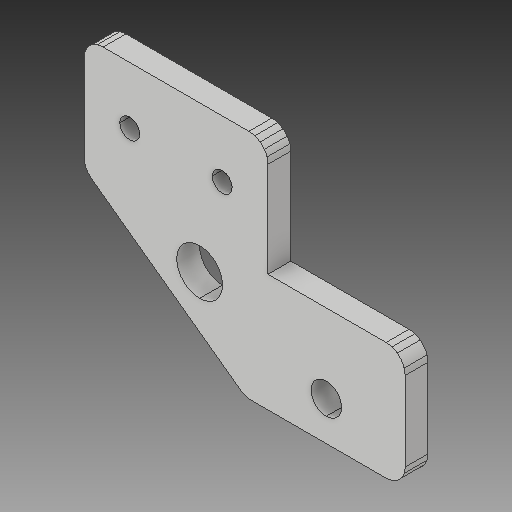
# Autodesk Inventor part: Leadscrew-rod-holder
Saved by Autodesk Inventor 2018 (Build 220112000, 112)
## iProperties
Created: 2016-07-23
Part Number: Leadscrew-rod-holder
Material: Generic
Document SubType Name: Modeling
Designer: joshm_000
Density: 1 g/cm^3
Appearance: Default
Author: joshm_000
Autodesk Inventor part; units mm, degrees
ref_plane "YZ Plane" through (0, 0, 0) normal (1, 0, 0) x (0, 1, 0)
ref_plane "XZ Plane" through (0, 0, 0) normal (0, 1, 0) x (-1, 0, 0)
ref_plane "XY Plane" through (0, 0, 0) normal (0, 0, 1) x (1, 0, 0)
sketch "Sketch1" plane through (0, 0, 0) normal (0, 0, 1) x (1, 0, 0)
  line L0 (83.1982, 140.877) -> (83.1982, 118.4214)
  spline S0 degree 3 poles (83.1982, 118.4214) (83.1982, 117.8956) (83.2805, 117.3761) (83.443, 116.8762) knots 1 1 1 1 2 2 2 2
  line L1 (83.1982, 118.4214) -> (83.1982, 117.8956) construction
  line L2 (83.1982, 117.8956) -> (83.2805, 117.3761) construction
  line L3 (83.2805, 117.3761) -> (83.443, 116.8762) construction
  spline S1 degree 3 poles (83.443, 116.8762) (83.6054, 116.3762) (83.8442, 115.9078) (84.1532, 115.4824) knots 2 2 2 2 3 3 3 3
  line L4 (83.443, 116.8762) -> (83.6054, 116.3762) construction
  line L5 (83.6054, 116.3762) -> (83.8442, 115.9078) construction
  line L6 (83.8442, 115.9078) -> (84.1532, 115.4824) construction
  spline S2 degree 3 poles (84.1532, 115.4824) (84.4612, 115.0586) (84.8315, 114.6879) (85.2551, 114.3792) knots 3 3 3 3 4 4 4 4
  line L7 (84.1532, 115.4824) -> (84.4612, 115.0586) construction
  line L8 (84.4612, 115.0586) -> (84.8315, 114.6879) construction
  line L9 (84.8315, 114.6879) -> (85.2551, 114.3792) construction
  line L10 (85.2551, 114.3792) -> (124.2313, 85.9985)
  spline S3 degree 3 poles (124.2313, 85.9985) (124.6565, 85.689) (125.1247, 85.4497) (125.6245, 85.2868) knots 5 5 5 5 6 6 6 6
  line L11 (124.2313, 85.9985) -> (124.6565, 85.689) construction
  line L12 (124.6565, 85.689) -> (125.1247, 85.4497) construction
  line L13 (125.1247, 85.4497) -> (125.6245, 85.2868) construction
  spline S4 degree 3 poles (125.6245, 85.2868) (126.1262, 85.1233) (126.647, 85.0405) (127.1745, 85.0405) knots 6 6 6 6 7 7 7 7
  line L14 (125.6245, 85.2868) -> (126.1262, 85.1233) construction
  line L15 (126.1262, 85.1233) -> (126.647, 85.0405) construction
  line L16 (126.647, 85.0405) -> (127.1745, 85.0405) construction
  line L17 (127.1745, 85.0405) -> (157.5604, 85.0405)
  line L18 (157.5604, 85.0405) -> (162.48, 85.0405)
  spline S5 degree 3 poles (162.48, 85.0405) (163.0057, 85.0405) (163.5251, 85.1228) (164.0251, 85.2852) (164.5252, 85.4477) (164.9935, 85.6864) (165.419, 85.9954) knots 9 9 9 9 10 10 10 11 11 11 11
  line L19 (162.48, 85.0405) -> (163.0057, 85.0405) construction
  line L20 (163.0057, 85.0405) -> (163.5251, 85.1228) construction
  line L21 (163.5251, 85.1228) -> (164.0251, 85.2852) construction
  line L22 (164.0251, 85.2852) -> (164.5252, 85.4477) construction
  line L23 (164.5252, 85.4477) -> (164.9935, 85.6864) construction
  line L24 (164.9935, 85.6864) -> (165.419, 85.9954) construction
  spline S6 degree 3 poles (165.419, 85.9954) (165.8443, 86.3045) (166.216, 86.6762) (166.5251, 87.1017) knots 11 11 11 11 12 12 12 12
  line L25 (165.419, 85.9954) -> (165.8443, 86.3045) construction
  line L26 (165.8443, 86.3045) -> (166.216, 86.6762) construction
  line L27 (166.216, 86.6762) -> (166.5251, 87.1017) construction
  spline S7 degree 3 poles (166.5251, 87.1017) (166.8341, 87.5268) (167.0728, 87.9953) (167.2353, 88.4955) knots 12 12 12 12 13 13 13 13
  line L28 (166.5251, 87.1017) -> (166.8341, 87.5268) construction
  line L29 (166.8341, 87.5268) -> (167.0728, 87.9953) construction
  line L30 (167.0728, 87.9953) -> (167.2353, 88.4955) construction
  spline S8 degree 3 poles (167.2353, 88.4955) (167.3977, 88.9954) (167.48, 89.5146) (167.48, 90.0403) knots 13 13 13 13 14 14 14 14
  line L31 (167.2353, 88.4955) -> (167.3977, 88.9954) construction
  line L32 (167.3977, 88.9954) -> (167.48, 89.5146) construction
  line L33 (167.48, 89.5146) -> (167.48, 90.0403) construction
  line L34 (167.48, 90.0403) -> (167.48, 110.877)
  spline S9 degree 3 poles (167.48, 110.877) (167.48, 111.4027) (167.3977, 111.9219) (167.2353, 112.4221) knots 15 15 15 15 16 16 16 16
  line L35 (167.48, 110.877) -> (167.48, 111.4027) construction
  line L36 (167.48, 111.4027) -> (167.3977, 111.9219) construction
  line L37 (167.3977, 111.9219) -> (167.2353, 112.4221) construction
  spline S10 degree 3 poles (167.2353, 112.4221) (167.0728, 112.9221) (166.8341, 113.3905) (166.5251, 113.816) (166.216, 114.2414) (165.8443, 114.6132) (165.419, 114.9222) knots 16 16 16 16 17 17 17 18 18 18 18
  line L38 (167.2353, 112.4221) -> (167.0728, 112.9221) construction
  line L39 (167.0728, 112.9221) -> (166.8341, 113.3905) construction
  line L40 (166.8341, 113.3905) -> (166.5251, 113.816) construction
  line L41 (166.5251, 113.816) -> (166.216, 114.2414) construction
  line L42 (166.216, 114.2414) -> (165.8443, 114.6132) construction
  line L43 (165.8443, 114.6132) -> (165.419, 114.9222) construction
  spline S11 degree 3 poles (165.419, 114.9222) (164.9935, 115.2312) (164.5252, 115.47) (164.0251, 115.6322) knots 18 18 18 18 19 19 19 19
  line L44 (165.419, 114.9222) -> (164.9935, 115.2312) construction
  line L45 (164.9935, 115.2312) -> (164.5252, 115.47) construction
  line L46 (164.5252, 115.47) -> (164.0251, 115.6322) construction
  spline S12 degree 3 poles (164.0251, 115.6322) (163.5251, 115.7948) (163.0057, 115.877) (162.48, 115.877) knots 19 19 19 19 20 20 20 20
  line L47 (164.0251, 115.6322) -> (163.5251, 115.7948) construction
  line L48 (163.5251, 115.7948) -> (163.0057, 115.877) construction
  line L49 (163.0057, 115.877) -> (162.48, 115.877) construction
  line L50 (162.48, 115.877) -> (131.48, 115.877)
  line L51 (131.48, 115.877) -> (131.48, 140.877)
  spline S13 degree 3 poles (131.48, 140.877) (131.48, 141.4029) (131.3978, 141.9221) (131.2352, 142.422) knots 22 22 22 22 23 23 23 23
  line L52 (131.48, 140.877) -> (131.48, 141.4029) construction
  line L53 (131.48, 141.4029) -> (131.3978, 141.9221) construction
  line L54 (131.3978, 141.9221) -> (131.2352, 142.422) construction
  spline S14 degree 3 poles (131.2352, 142.422) (131.073, 142.9222) (130.8342, 143.3906) (130.5252, 143.8159) knots 23 23 23 23 24 24 24 24
  line L55 (131.2352, 142.422) -> (131.073, 142.9222) construction
  line L56 (131.073, 142.9222) -> (130.8342, 143.3906) construction
  line L57 (130.8342, 143.3906) -> (130.5252, 143.8159) construction
  spline S15 degree 3 poles (130.5252, 143.8159) (130.2162, 144.2413) (129.8443, 144.6131) (129.419, 144.9221) knots 24 24 24 24 25 25 25 25
  line L58 (130.5252, 143.8159) -> (130.2162, 144.2413) construction
  line L59 (130.2162, 144.2413) -> (129.8443, 144.6131) construction
  line L60 (129.8443, 144.6131) -> (129.419, 144.9221) construction
  spline S16 degree 3 poles (129.419, 144.9221) (128.9935, 145.2311) (128.5251, 145.4698) (128.0251, 145.6325) knots 25 25 25 25 26 26 26 26
  line L61 (129.419, 144.9221) -> (128.9935, 145.2311) construction
  line L62 (128.9935, 145.2311) -> (128.5251, 145.4698) construction
  line L63 (128.5251, 145.4698) -> (128.0251, 145.6325) construction
  spline S17 degree 3 poles (128.0251, 145.6325) (127.525, 145.7947) (127.0057, 145.8771) (126.48, 145.8771) knots 26 26 26 26 27 27 27 27
  line L64 (128.0251, 145.6325) -> (127.525, 145.7947) construction
  line L65 (127.525, 145.7947) -> (127.0057, 145.8771) construction
  line L66 (127.0057, 145.8771) -> (126.48, 145.8771) construction
  line L67 (126.48, 145.8771) -> (120.08, 145.8771)
  line L68 (120.08, 145.8771) -> (115.1604, 145.8771)
  line L69 (115.1604, 145.8771) -> (88.1982, 145.8771)
  spline S18 degree 3 poles (88.1982, 145.8771) (87.6723, 145.8771) (87.1532, 145.7947) (86.6533, 145.6325) knots 30 30 30 30 31 31 31 31
  line L70 (88.1982, 145.8771) -> (87.6723, 145.8771) construction
  line L71 (87.6723, 145.8771) -> (87.1532, 145.7947) construction
  line L72 (87.1532, 145.7947) -> (86.6533, 145.6325) construction
  spline S19 degree 3 poles (86.6533, 145.6325) (86.1531, 145.4698) (85.6845, 145.2311) (85.2594, 144.9221) knots 31 31 31 31 32 32 32 32
  line L73 (86.6533, 145.6325) -> (86.1531, 145.4698) construction
  line L74 (86.1531, 145.4698) -> (85.6845, 145.2311) construction
  line L75 (85.6845, 145.2311) -> (85.2594, 144.9221) construction
  spline S20 degree 3 poles (85.2594, 144.9221) (84.8339, 144.6131) (84.4622, 144.2413) (84.1532, 143.8159) knots 32 32 32 32 33 33 33 33
  line L76 (85.2594, 144.9221) -> (84.8339, 144.6131) construction
  line L77 (84.8339, 144.6131) -> (84.4622, 144.2413) construction
  line L78 (84.4622, 144.2413) -> (84.1532, 143.8159) construction
  spline S21 degree 3 poles (84.1532, 143.8159) (83.8442, 143.3906) (83.6054, 142.9222) (83.443, 142.422) knots 33 33 33 33 34 34 34 34
  line L79 (84.1532, 143.8159) -> (83.8442, 143.3906) construction
  line L80 (83.8442, 143.3906) -> (83.6054, 142.9222) construction
  line L81 (83.6054, 142.9222) -> (83.443, 142.422) construction
  spline S22 degree 3 poles (83.443, 142.422) (83.2805, 141.9221) (83.1982, 141.4029) (83.1982, 140.877) knots 34 34 34 34 35 35 35 35
  line L82 (83.443, 142.422) -> (83.2805, 141.9221) construction
  line L83 (83.2805, 141.9221) -> (83.1982, 141.4029) construction
  line L84 (83.1982, 141.4029) -> (83.1982, 140.877) construction
  spline S23 degree 3 poles (146.7912, 91.2547) (144.5819, 91.2547) (142.7911, 93.0455) (142.7911, 95.2547) (142.7911, 97.4638) (144.5819, 99.2546) (146.7912, 99.2546) (149.0002, 99.2546) (150.7911, 97.4638) (150.7911, 95.2547) (150.7911, 93.0455) (149.0002, 91.2547) (146.7912, 91.2547) knots 0 0 0 0 1 1 1 2 2 2 3 3 3 4 4 4 4
  line L85 (146.7912, 91.2547) -> (144.5819, 91.2547) construction
  line L86 (144.5819, 91.2547) -> (142.7911, 93.0455) construction
  line L87 (142.7911, 93.0455) -> (142.7911, 95.2547) construction
  line L88 (142.7911, 95.2547) -> (142.7911, 97.4638) construction
  line L89 (142.7911, 97.4638) -> (144.5819, 99.2546) construction
  line L90 (144.5819, 99.2546) -> (146.7912, 99.2546) construction
  line L91 (146.7912, 99.2546) -> (149.0002, 99.2546) construction
  line L92 (149.0002, 99.2546) -> (150.7911, 97.4638) construction
  line L93 (150.7911, 97.4638) -> (150.7911, 95.2547) construction
  line L94 (150.7911, 95.2547) -> (150.7911, 93.0455) construction
  line L95 (150.7911, 93.0455) -> (149.0002, 91.2547) construction
  line L96 (149.0002, 91.2547) -> (146.7912, 91.2547) construction
  spline S24 degree 3 poles (95.1982, 128.2771) (93.7622, 128.2771) (92.5981, 129.4412) (92.5981, 130.8771) (92.5981, 132.313) (93.7622, 133.4771) (95.1982, 133.4771) (96.6341, 133.4771) (97.7982, 132.313) (97.7982, 130.8771) (97.7982, 129.4412) (96.6341, 128.2771) (95.1982, 128.2771) knots 0 0 0 0 1 1 1 2 2 2 3 3 3 4 4 4 4
  line L97 (95.1982, 128.2771) -> (93.7622, 128.2771) construction
  line L98 (93.7622, 128.2771) -> (92.5981, 129.4412) construction
  line L99 (92.5981, 129.4412) -> (92.5981, 130.8771) construction
  line L100 (92.5981, 130.8771) -> (92.5981, 132.313) construction
  line L101 (92.5981, 132.313) -> (93.7622, 133.4771) construction
  line L102 (93.7622, 133.4771) -> (95.1982, 133.4771) construction
  line L103 (95.1982, 133.4771) -> (96.6341, 133.4771) construction
  line L104 (96.6341, 133.4771) -> (97.7982, 132.313) construction
  line L105 (97.7982, 132.313) -> (97.7982, 130.8771) construction
  line L106 (97.7982, 130.8771) -> (97.7982, 129.4412) construction
  line L107 (97.7982, 129.4412) -> (96.6341, 128.2771) construction
  line L108 (96.6341, 128.2771) -> (95.1982, 128.2771) construction
  spline S25 degree 3 poles (119.48, 128.2771) (118.044, 128.2771) (116.88, 129.4412) (116.88, 130.8771) (116.88, 132.313) (118.044, 133.4771) (119.48, 133.4771) (120.916, 133.4771) (122.0799, 132.313) (122.0799, 130.8771) (122.0799, 129.4412) (120.916, 128.2771) (119.48, 128.2771) knots 0 0 0 0 1 1 1 2 2 2 3 3 3 4 4 4 4
  line L109 (119.48, 128.2771) -> (118.044, 128.2771) construction
  line L110 (118.044, 128.2771) -> (116.88, 129.4412) construction
  line L111 (116.88, 129.4412) -> (116.88, 130.8771) construction
  line L112 (116.88, 130.8771) -> (116.88, 132.313) construction
  line L113 (116.88, 132.313) -> (118.044, 133.4771) construction
  line L114 (118.044, 133.4771) -> (119.48, 133.4771) construction
  line L115 (119.48, 133.4771) -> (120.916, 133.4771) construction
  line L116 (120.916, 133.4771) -> (122.0799, 132.313) construction
  line L117 (122.0799, 132.313) -> (122.0799, 130.8771) construction
  line L118 (122.0799, 130.8771) -> (122.0799, 129.4412) construction
  line L119 (122.0799, 129.4412) -> (120.916, 128.2771) construction
  line L120 (120.916, 128.2771) -> (119.48, 128.2771) construction
  spline S26 degree 3 poles (146.7912, 91.5045) (144.72, 91.5045) (143.0412, 93.1836) (143.0412, 95.2547) (143.0412, 97.3257) (144.72, 99.0045) (146.7912, 99.0045) (148.8622, 99.0045) (150.5412, 97.3257) (150.5412, 95.2547) (150.5412, 93.1836) (148.8622, 91.5045) (146.7912, 91.5045) knots 0 0 0 0 1 1 1 2 2 2 3 3 3 4 4 4 4
  line L121 (146.7912, 91.5045) -> (144.72, 91.5045) construction
  line L122 (144.72, 91.5045) -> (143.0412, 93.1836) construction
  line L123 (143.0412, 93.1836) -> (143.0412, 95.2547) construction
  line L124 (143.0412, 95.2547) -> (143.0412, 97.3257) construction
  line L125 (143.0412, 97.3257) -> (144.72, 99.0045) construction
  line L126 (144.72, 99.0045) -> (146.7912, 99.0045) construction
  line L127 (146.7912, 99.0045) -> (148.8622, 99.0045) construction
  line L128 (148.8622, 99.0045) -> (150.5412, 97.3257) construction
  line L129 (150.5412, 97.3257) -> (150.5412, 95.2547) construction
  line L130 (150.5412, 95.2547) -> (150.5412, 93.1836) construction
  line L131 (150.5412, 93.1836) -> (148.8622, 91.5045) construction
  line L132 (148.8622, 91.5045) -> (146.7912, 91.5045) construction
  spline S27 degree 3 poles (113.5312, 101.426) (110.2174, 101.426) (107.5312, 104.1123) (107.5312, 107.426) (107.5312, 110.7398) (110.2174, 113.426) (113.5312, 113.426) (116.8449, 113.426) (119.5312, 110.7398) (119.5312, 107.426) (119.5312, 104.1123) (116.8449, 101.426) (113.5312, 101.426) knots 0 0 0 0 1 1 1 2 2 2 3 3 3 4 4 4 4
  line L133 (113.5312, 101.426) -> (110.2174, 101.426) construction
  line L134 (110.2174, 101.426) -> (107.5312, 104.1123) construction
  line L135 (107.5312, 104.1123) -> (107.5312, 107.426) construction
  line L136 (107.5312, 107.426) -> (107.5312, 110.7398) construction
  line L137 (107.5312, 110.7398) -> (110.2174, 113.426) construction
  line L138 (110.2174, 113.426) -> (113.5312, 113.426) construction
  line L139 (113.5312, 113.426) -> (116.8449, 113.426) construction
  line L140 (116.8449, 113.426) -> (119.5312, 110.7398) construction
  line L141 (119.5312, 110.7398) -> (119.5312, 107.426) construction
  line L142 (119.5312, 107.426) -> (119.5312, 104.1123) construction
  line L143 (119.5312, 104.1123) -> (116.8449, 101.426) construction
  line L144 (116.8449, 101.426) -> (113.5312, 101.426) construction
  point P0 (0, 0)
  constraints: 20 end point, 79 other
extrude "Extrusion1" add sketch "Sketch1" along normal blind 6 contours S22 S21 S20 S19 S18 L69 L68 L67 S17 S16 S15 S14 S13 L51 L50 S12 S11 S10 S9 L34 S8 S7 S6 S5 L18 L17 S4 S3 L10 S2 S1 S0 L0
sketch "Sketch2" plane through (0, 0, 0) normal (0, 0, -1) x (-1, 0, 0)
  line L0 (-83.1982, 140.877) -> (-83.1982, 118.4214) projected
  line L1 (-126.48, 145.8771) -> (-88.1982, 145.8771) projected
  line L2 (-131.48, 115.877) -> (-131.48, 140.877) projected
  line L3 (-162.48, 115.877) -> (-131.48, 115.877) projected
  line L4 (-167.48, 90.0403) -> (-167.48, 110.877) projected
  line L5 (-127.1745, 85.0405) -> (-162.48, 85.0405) projected
  line L6 (-85.2551, 114.3792) -> (-124.2313, 85.9985) projected
  line L7 (-92.5981, 130.874) -> (-97.7982, 130.874)
  line L8 (-116.88, 130.874) -> (-122.0799, 130.874)
  point P0 (0, 0)
  point P1 (-113.5312, 101.426)
  point P2 (-146.7912, 91.2547)
  point P3 (-95.1982, 128.2771)
  point P4 (-119.48, 128.2771)
  point P5 (-83.443, 116.8762)
  point P6 (-83.443, 142.422)
  point P7 (-84.1532, 143.8159)
  point P8 (-85.2594, 144.9221)
  point P9 (-86.6533, 145.6325)
  point P10 (-128.0251, 145.6325)
  point P11 (-129.419, 144.9221)
  point P12 (-130.5252, 143.8159)
  point P13 (-131.2352, 142.422)
  point P14 (-164.0251, 115.6322)
  point P15 (-165.419, 114.9222)
  point P16 (-167.2353, 112.4221)
  point P17 (-167.2353, 88.4955)
  point P18 (-166.5251, 87.1017)
  point P19 (-165.419, 85.9954)
  point P20 (-125.6245, 85.2868)
  point P21 (-84.1532, 115.4824)
  point P22 (-95.1982, 130.874)
  point P23 (-119.48, 130.874)
  constraints: 4 end point, 2 midpoint, 2 point on line, 1 horizontal, 31 other
hole "Hole1" at (95.1982, 130.874, 0) at (119.48, 130.874, 0) direction (0, 0, 1) diameter 5.2 end through all
body "Solid1"
